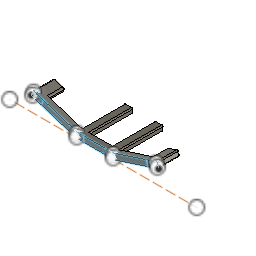
Book holder (Autodesk Fusion 360 design; units mm, degrees)
Autodesk Fusion 360 part; units mm, degrees
sketch "Sketch1" plane through (0, 0, 0) normal (0, 1, 0) x (1, 0, 0)
  line L0 (-49.947773, -20.432475) -> (20.052227, -20.432475)
  line L1 (20.052227, -20.432475) -> (98.989918, -46.080886)
  line L2 (20.052227, -20.432475) -> (170, -20.432475) construction
  line L3 (-49.947773, -20.432475) -> (-128.885463, -46.080886)
  line L4 (-49.947773, -20.432475) -> (-170, -20.432475) construction
  line L5 (-48.363928, -30.432475) -> (-125.795293, -55.591451)
  line L6 (-48.363928, -30.432475) -> (18.468383, -30.432475)
  line L7 (18.468383, -30.432475) -> (95.899748, -55.591451)
  line L8 (-128.31544, -54.307372) -> (-130.169542, -48.601033)
  line L9 (98.419895, -54.307372) -> (100.273997, -48.601033)
  line L10 (78.780731, -50.029145) -> (81.870901, -40.51858)
  line L11 (-108.676276, -50.029145) -> (-111.766446, -40.51858)
  arc A0 (-128.31544, -54.307372) -> (-125.795293, -55.591451) centre (-126.413327, -53.689338) ccw
  arc A1 (-128.885463, -46.080886) -> (-130.169542, -48.601033) centre (-128.267429, -47.982999) ccw
  line L12 (-47.947773, -20.432475) -> (-34.947773, -20.432475)
  line L13 (-34.947773, -20.432475) -> (-34.947773, -30.432475)
  line L14 (-34.947773, -30.432475) -> (-47.947773, -30.432475)
  line L15 (-49.947773, -28.432475) -> (-49.947773, -22.432475)
  line L16 (18.052227, -20.432475) -> (5.052227, -20.432475)
  line L17 (5.052227, -20.432475) -> (5.052227, -30.432475)
  line L18 (5.052227, -30.432475) -> (18.052227, -30.432475)
  line L19 (20.052227, -28.432475) -> (20.052227, -22.432475)
  arc A2 (18.052227, -30.432475) -> (20.052227, -28.432475) centre (18.052227, -28.432475) ccw
  arc A3 (20.052227, -22.432475) -> (18.052227, -20.432475) centre (18.052227, -22.432475) ccw
  arc A4 (-49.947773, -28.432475) -> (-47.947773, -30.432475) centre (-47.947773, -28.432475) ccw
  arc A5 (-47.947773, -20.432475) -> (-49.947773, -22.432475) centre (-47.947773, -22.432475) ccw
  arc A6 (95.899748, -55.591451) -> (98.419895, -54.307372) centre (96.517782, -53.689338) ccw
  arc A7 (100.273997, -48.601033) -> (98.989918, -46.080886) centre (98.371884, -47.982999) ccw
  point P0 (100.892031, -46.69892)
  point P1 (-130.787576, -46.69892)
  dimension "d1" = 70
  dimension "d2" = 85
  dimension "d3" = 18
  dimension "d4" = 18
  dimension "d5" = 85
  dimension "d9" = 2
  dimension "d10" = 15
  dimension "d11" = 15
  dimension "d12" = 2
  dimension "d13" = 2
  dimension "d14" = 2
  constraint horizontal L0
  constraint horizontal L2
  constraint horizontal L4
  constraint perpendicular L3 L8
  constraint perpendicular L1 L9
  constraint tangent L5 A0
  constraint tangent L8 A0
  constraint tangent L3 A1
  constraint tangent L8 A1
  constraint equal A0 A1
  constraint horizontal L12
  constraint vertical L13
  constraint horizontal L14
  constraint vertical L15
  constraint horizontal L16
  constraint vertical L17
  constraint horizontal L18
  constraint vertical L19
  constraint tangent L18 A2
  constraint tangent L19 A2
  constraint tangent L19 A3
  constraint tangent L16 A3
  constraint equal A2 A3
  constraint tangent L14 A4
  constraint tangent L15 A4
  constraint tangent L15 A5
  constraint tangent L12 A5
  constraint equal A4 A5
  constraint tangent L7 A6
  constraint tangent L9 A6
  constraint tangent L9 A7
  constraint tangent L1 A7
  constraint equal A6 A7
  measures "d3" angle of L1 L2
  measures "d4" angle of L3 L4
  measures "d9" radius of A0
  measures "d12" radius of A2
  measures "d13" radius of A4
  measures "d14" radius of A6
extrude "Extrude1" add sketch "Sketch1" along normal blind 10 contours L0 L3 L5 L6 L11 L15 A4 A5 | L0 L6 L12 L13 L14 L15 A4 A5 | L3 L5 L8 L11 A0 A1 | L0 L6 L13 L17 | L0 L6 L16 L17 L18 L19 A2 A3 | L0 L1 L6 L7 L10 L19 A2 A3 | L1 L7 L9 L10 A6 A7 picked at (-90.10316, -39.847889) picked at (-39.281106, -27.099142) picked at (-116.442729, -45.54287) picked at (-8.281106, -27.099142) picked at (13.718894, -27.099142) picked at (60.207615, -39.847889) picked at (86.547183, -45.54287)
extrude "Extrude2" add sketch "Sketch1" along normal blind 90 contours L0 L6 L12 L13 L14 L15 A4 A5 | L0 L6 L16 L17 L18 L19 A2 A3 picked at (-39.281106, -27.099142) picked at (13.718894, -27.099142)
extrude "Extrude3" add sketch "Sketch1" along normal blind 40 contours L3 L5 L8 L11 A0 A1 | L1 L7 L9 L10 A6 A7 picked at (-116.442729, -45.54287) picked at (86.547183, -45.54287)
fillet "Fillet1" radius 2 1 edges at (-110.221361, 40, 45.273863)
fillet "Fillet2" radius 3 9 edges at (-111.766446, 24, 40.51858) (-112.323562, 39.414214, 40.699598) (-121.277011, 40, 43.60875) (-130.049442, 40, 47.075018) (-129.242491, 40, 51.454202) (-127.321308, 40, 55.471351) (-118.186841, 40, 53.119315) (-109.233392, 39.414214, 50.210163) (-108.676276, 24, 50.029145)
fillet "Fillet3" radius 2 1 edges at (81.870901, 25, 40.51858)
fillet "Fillet4" radius 2 1 edges at (78.780731, 25, 50.029145)
fillet "Fillet5" radius 3 8 edges at (99.346946, 40, 51.454202) (100.153897, 40, 47.075018) (91.381466, 40, 43.60875) (82.246999, 40, 41.256714) (80.325816, 40, 45.273863) (79.518865, 40, 49.653047) (88.291296, 40, 53.119315) (97.425763, 40, 55.471351)
fillet "Fillet6" radius 2 1 edges at (-34.947773, 50, 20.432475)
fillet "Fillet6" radius 2 1 edges at (-34.947773, 50, 30.432475)
fillet "Fillet6" radius 2 2 edges at (5.052227, 50, 20.432475) (5.052227, 50, 30.432475)
fillet "Fillet7" radius 2 8 edges at (-49.947773, 90, 25.432475) (-49.361986, 90, 29.846689) (-42.447773, 90, 30.432475) (-35.533559, 90, 29.846689) (-34.947773, 90, 25.432475) (-35.533559, 90, 21.018262) (-42.447773, 90, 20.432475) (-49.361986, 90, 21.018262)
fillet "Fillet7" radius 2 8 edges at (20.052227, 90, 25.432475) (19.466441, 90, 21.018262) (12.552227, 90, 20.432475) (5.638014, 90, 21.018262) (5.052227, 90, 25.432475) (5.638014, 90, 29.846689) (12.552227, 90, 30.432475) (19.466441, 90, 29.846689)
